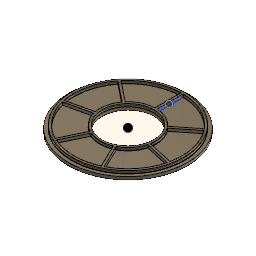
router_table_insert_v1 (Autodesk Fusion 360 design; units mm, degrees)
Autodesk Fusion 360 part; units mm, degrees
note: some values were not read from the file. Set by a fixed rule: which sketch regions a step uses.
sketch "Sketch1" plane through (0, 0, 0) normal (0, 1, 0) x (1, 0, 0)
  circle A0 centre (0, 0) radius 48.6
  circle A1 centre (0, 0) radius 21
  dimension "d1" = 97.2
  dimension "d7" = 42
  measures "d1" diameter of A0
  measures "d7" diameter of A1
extrude "Extrude1" add sketch "Sketch1" along normal blind 2.5
sketch "support_ribs" plane through (0, 2.5, 0) normal (0, 1, 0) x (-1, 0, 0)
  circle A0 centre (0, 0) radius 21
  circle A1 centre (0, 0) radius 48.6
  circle A2 centre (0, 0) radius 45.8
  circle A3 centre (0, 0) radius 44
  circle A4 centre (0, 0) radius 21
  circle A5 centre (0, 0) radius 22.8
  line L0 (-0.9352, -21.9) -> (0.8648, -21.9)
  line L1 (0.8648, -21.9) -> (0.8648, -44.9)
  line L2 (0.8648, -44.9) -> (-0.9352, -44.9)
  line L3 (-0.9352, -44.9) -> (-0.9352, -21.9)
  line L4 (-0.9352, -21.9) -> (0.8648, -44.9) construction
  line L5 (0.8648, -21.9) -> (-0.9352, -44.9) construction
  dimension "d12" = 91.6
  dimension "d13" = 88
  dimension "d14" = 42
  dimension "d15" = 45.6
  dimension "d16" = 33.4
  dimension "d17" = 1.8
  dimension "d18" = 23
  measures "d12" diameter of A2
  measures "d13" diameter of A3
  measures "d14" diameter of A4
  measures "d15" diameter of A5
  measures "d16" distance of A0.centre
extrude "Extrude2" add sketch "support_ribs" along normal blind 2.3 contours A2 | A3 L1 L2 L3 | A5 L0 L1 L3 | A5 L0 L1 L3
extrude "Extrude3" add sketch "support_ribs" along normal blind 2.3 contours A3 A5 L1 L3 picked at (0.6649, -29.8579)
pattern_circular "C-Pattern1" count 7 over 360 about axis through (0, 1.75, 0) along (0, 1, 0) of "Extrude3"
equation "d1 = insert_dia"
equation "insert_dia = 97.2 mm"
equation "bit_dia = 30 mm"
equation "bit_clearance = 6 mm" comment "clearance between bit and insert"
equation "insert_thick = 2.5 mm"
equation "support_rib_height = 2.3 mm"
equation "d7 = bit_dia + bit_clearance * 2"
equation "d8 = insert_thick"
equation "insert_lip = 2.8 mm"
equation "support_rib_width = 1.8 mm"
equation "d12 = insert_dia - 2 * insert_lip"
equation "d13 = insert_dia - 2 * insert_lip - support_rib_width * 2"
equation "d14 = bit_dia + 2 * bit_clearance"
equation "d15 = bit_dia + 2 * bit_clearance + 2 * support_rib_width"
equation "d16 = ( insert_dia - 2 * insert_lip - ( bit_dia + 2 * bit_clearance ) ) / 4 + bit_dia / 2 + bit_clearance"
equation "d17 = support_rib_width"
equation "d18 = insert_dia / 2 - insert_lip - bit_dia / 2 - bit_clearance - support_rib_width"
equation "d19 = support_rib_height"
equation "d21 = support_rib_height"
